Autodesk Inventor part; units mm, degrees
(part 4 of 6)
  line L2631 (12.0453, 185.408) -> (12.0771, 185.6164)
  line L2632 (12.0771, 185.6164) -> (12.1288, 185.8178)
  line L2633 (12.1288, 185.8178) -> (12.1994, 186.0107)
  line L2634 (12.1994, 186.0107) -> (12.288, 186.1941)
  line L2635 (12.288, 186.1941) -> (12.393, 186.3673)
  line L2636 (12.393, 186.3673) -> (12.514, 186.529)
  line L2637 (12.514, 186.529) -> (12.6495, 186.6782)
  line L2638 (12.6495, 186.6782) -> (12.7987, 186.8137)
  line L2639 (12.7987, 186.8137) -> (12.9603, 186.9345)
  line L2640 (12.9603, 186.9345) -> (13.1334, 187.0397)
  line L2641 (13.1334, 187.0397) -> (13.317, 187.1281)
  line L2642 (13.317, 187.1281) -> (13.5099, 187.1987)
  line L2643 (13.5099, 187.1987) -> (13.7111, 187.2506)
  line L2644 (13.7111, 187.2506) -> (13.9197, 187.2823)
  line L2645 (13.9197, 187.2823) -> (14.1344, 187.2931)
  line L2646 (14.1344, 187.2931) -> (14.3492, 187.2823)
  line L2647 (14.3492, 187.2823) -> (14.5576, 187.2506)
  line L2648 (14.5576, 187.2506) -> (14.759, 187.1987)
  line L2649 (14.759, 187.1987) -> (14.9519, 187.1281)
  line L2650 (14.9519, 187.1281) -> (15.1355, 187.0397)
  line L2651 (15.1355, 187.0397) -> (15.3086, 186.9345)
  line L2652 (15.3086, 186.9345) -> (15.4702, 186.8137)
  line L2653 (15.4702, 186.8137) -> (15.6194, 186.6782)
  line L2654 (15.6194, 186.6782) -> (15.7549, 186.529)
  line L2655 (15.7549, 186.529) -> (15.8759, 186.3673)
  line L2656 (15.8759, 186.3673) -> (15.9809, 186.1941)
  line L2657 (15.9809, 186.1941) -> (16.0695, 186.0107)
  line L2658 (16.0695, 186.0107) -> (16.1401, 185.8178)
  line L2659 (16.1401, 185.8178) -> (16.1918, 185.6164)
  line L2660 (16.1918, 185.6164) -> (16.2236, 185.408)
  line L2661 (16.2236, 185.408) -> (16.2345, 185.1932)
  line L2662 (16.2345, 185.1932) -> (16.2236, 184.9785)
  line L2663 (16.2236, 184.9785) -> (16.1918, 184.7699)
  line L2664 (16.1918, 184.7699) -> (16.1401, 184.5688)
  line L2665 (16.1401, 184.5688) -> (16.0695, 184.3758)
  line L2666 (16.0695, 184.3758) -> (15.9809, 184.1922)
  line L2667 (15.9809, 184.1922) -> (15.8759, 184.0191)
  line L2668 (15.8759, 184.0191) -> (15.7549, 183.8573)
  line L2669 (15.7549, 183.8573) -> (15.6194, 183.7083)
  line L2670 (15.6194, 183.7083) -> (15.4702, 183.5728)
  line L2671 (15.4702, 183.5728) -> (15.3086, 183.4519)
  line L2672 (15.3086, 183.4519) -> (15.1355, 183.3466)
  line L2673 (15.1355, 183.3466) -> (14.9519, 183.2582)
  line L2674 (14.9519, 183.2582) -> (14.759, 183.1876)
  line L2675 (14.759, 183.1876) -> (14.5576, 183.1359)
  line L2676 (14.5576, 183.1359) -> (14.3492, 183.1041)
  line L2677 (14.3492, 183.1041) -> (14.1344, 183.0932)
  line L2678 (14.1344, 183.0932) -> (13.9197, 183.1041)
  line L2679 (13.9197, 183.1041) -> (13.7111, 183.1359)
  line L2680 (13.7111, 183.1359) -> (13.5099, 183.1876)
  line L2681 (13.5099, 183.1876) -> (13.317, 183.2582)
  line L2682 (13.317, 183.2582) -> (13.1334, 183.3466)
  line L2683 (13.1334, 183.3466) -> (12.9603, 183.4519)
  line L2684 (12.9603, 183.4519) -> (12.7987, 183.5728)
  line L2685 (12.7987, 183.5728) -> (12.6495, 183.7083)
  line L2686 (12.6495, 183.7083) -> (12.514, 183.8573)
  line L2687 (12.514, 183.8573) -> (12.393, 184.0191)
  line L2688 (12.393, 184.0191) -> (12.288, 184.1922)
  line L2689 (12.288, 184.1922) -> (12.1994, 184.3758)
  line L2690 (12.1994, 184.3758) -> (12.1288, 184.5688)
  line L2691 (12.1288, 184.5688) -> (12.0771, 184.7699)
  line L2692 (12.0771, 184.7699) -> (12.0453, 184.9785)
  line L2693 (12.0453, 184.9785) -> (12.0344, 185.1932)
  spline S7 degree 3 poles (8.728, 122.2027) (8.728, 119.9937) (10.5189, 118.2029) (12.7281, 118.2029) knots 0 0 0 0 1 1 1 1
  line L2694 (8.728, 122.2027) -> (8.728, 119.9937) construction
  line L2695 (8.728, 119.9937) -> (10.5189, 118.2029) construction
  line L2696 (10.5189, 118.2029) -> (12.7281, 118.2029) construction
  line L2697 (12.7281, 118.2029) -> (42.201, 118.2029)
  spline S8 degree 3 poles (42.201, 118.2029) (44.4102, 118.2029) (46.201, 119.9937) (46.201, 122.2027) knots 2 2 2 2 3 3 3 3
  line L2698 (42.201, 118.2029) -> (44.4102, 118.2029) construction
  line L2699 (44.4102, 118.2029) -> (46.201, 119.9937) construction
  line L2700 (46.201, 119.9937) -> (46.201, 122.2027) construction
  line L2701 (46.201, 122.2027) -> (46.201, 175.1969)
  spline S9 degree 3 poles (46.201, 175.1969) (46.201, 177.4059) (44.4102, 179.1968) (42.201, 179.1968) knots 4 4 4 4 5 5 5 5
  line L2702 (46.201, 175.1969) -> (46.201, 177.4059) construction
  line L2703 (46.201, 177.4059) -> (44.4102, 179.1968) construction
  line L2704 (44.4102, 179.1968) -> (42.201, 179.1968) construction
  line L2705 (42.201, 179.1968) -> (12.7281, 179.1968)
  spline S10 degree 3 poles (12.7281, 179.1968) (10.5189, 179.1968) (8.728, 177.4059) (8.728, 175.1969) knots 6 6 6 6 7 7 7 7
  line L2706 (12.7281, 179.1968) -> (10.5189, 179.1968) construction
  line L2707 (10.5189, 179.1968) -> (8.728, 177.4059) construction
  line L2708 (8.728, 177.4059) -> (8.728, 175.1969) construction
  line L2709 (8.728, 175.1969) -> (8.728, 122.2027)
  line L2710 (95.0822, 167.9448) -> (83.8302, 179.1968)
  line L2711 (83.8302, 179.1968) -> (61.6093, 179.1968)
  spline S11 degree 3 poles (61.6093, 179.1968) (59.4002, 179.1968) (57.6092, 177.4059) (57.6092, 175.1969) knots 2 2 2 2 3 3 3 3
  line L2712 (61.6093, 179.1968) -> (59.4002, 179.1968) construction
  line L2713 (59.4002, 179.1968) -> (57.6092, 177.4059) construction
  line L2714 (57.6092, 177.4059) -> (57.6092, 175.1969) construction
  line L2715 (57.6092, 175.1969) -> (57.6092, 122.2027)
  spline S12 degree 3 poles (57.6092, 122.2027) (57.6092, 119.9937) (59.4002, 118.2029) (61.6093, 118.2029) knots 4 4 4 4 5 5 5 5
  line L2716 (57.6092, 122.2027) -> (57.6092, 119.9937) construction
  line L2717 (57.6092, 119.9937) -> (59.4002, 118.2029) construction
  line L2718 (59.4002, 118.2029) -> (61.6093, 118.2029) construction
  line L2719 (61.6093, 118.2029) -> (91.0823, 118.2029)
  spline S13 degree 3 poles (91.0823, 118.2029) (93.2915, 118.2029) (95.0822, 119.9937) (95.0822, 122.2027) knots 6 6 6 6 7 7 7 7
  line L2720 (91.0823, 118.2029) -> (93.2915, 118.2029) construction
  line L2721 (93.2915, 118.2029) -> (95.0822, 119.9937) construction
  line L2722 (95.0822, 119.9937) -> (95.0822, 122.2027) construction
  line L2723 (95.0822, 122.2027) -> (95.0822, 167.9448)
  spline S14 degree 3 poles (98.6277, 167.2363) (98.6277, 164.4749) (100.8664, 162.2363) (103.6278, 162.2363) knots 0 0 0 0 1 1 1 1
  line L2724 (98.6277, 167.2363) -> (98.6277, 164.4749) construction
  line L2725 (98.6277, 164.4749) -> (100.8664, 162.2363) construction
  line L2726 (100.8664, 162.2363) -> (103.6278, 162.2363) construction
  line L2727 (103.6278, 162.2363) -> (106.6278, 162.2363)
  spline S15 degree 3 poles (106.6278, 162.2363) (109.3894, 162.2363) (111.6276, 164.4749) (111.6276, 167.2363) knots 2 2 2 2 3 3 3 3
  line L2728 (106.6278, 162.2363) -> (109.3894, 162.2363) construction
  line L2729 (109.3894, 162.2363) -> (111.6276, 164.4749) construction
  line L2730 (111.6276, 164.4749) -> (111.6276, 167.2363) construction
  line L2731 (111.6276, 167.2363) -> (111.6276, 174.2373)
  spline S16 degree 3 poles (111.6276, 174.2373) (111.6276, 176.9987) (109.3894, 179.2373) (106.6278, 179.2373) knots 4 4 4 4 5 5 5 5
  line L2732 (111.6276, 174.2373) -> (111.6276, 176.9987) construction
  line L2733 (111.6276, 176.9987) -> (109.3894, 179.2373) construction
  line L2734 (109.3894, 179.2373) -> (106.6278, 179.2373) construction
  line L2735 (106.6278, 179.2373) -> (103.6278, 179.2373)
  spline S17 degree 3 poles (103.6278, 179.2373) (100.8664, 179.2373) (98.6277, 176.9987) (98.6277, 174.2373) knots 6 6 6 6 7 7 7 7
  line L2736 (103.6278, 179.2373) -> (100.8664, 179.2373) construction
  line L2737 (100.8664, 179.2373) -> (98.6277, 176.9987) construction
  line L2738 (98.6277, 176.9987) -> (98.6277, 174.2373) construction
  line L2739 (98.6277, 174.2373) -> (98.6277, 167.2363)
  spline S18 degree 3 poles (98.6277, 145.2363) (98.6277, 142.475) (100.8664, 140.2364) (103.6278, 140.2364) knots 0 0 0 0 1 1 1 1
  line L2740 (98.6277, 145.2363) -> (98.6277, 142.475) construction
  line L2741 (98.6277, 142.475) -> (100.8664, 140.2364) construction
  line L2742 (100.8664, 140.2364) -> (103.6278, 140.2364) construction
  line L2743 (103.6278, 140.2364) -> (106.6278, 140.2364)
  spline S19 degree 3 poles (106.6278, 140.2364) (109.3894, 140.2364) (111.6276, 142.475) (111.6276, 145.2363) knots 2 2 2 2 3 3 3 3
  line L2744 (106.6278, 140.2364) -> (109.3894, 140.2364) construction
  line L2745 (109.3894, 140.2364) -> (111.6276, 142.475) construction
  line L2746 (111.6276, 142.475) -> (111.6276, 145.2363) construction
  line L2747 (111.6276, 145.2363) -> (111.6276, 152.2374)
  spline S20 degree 3 poles (111.6276, 152.2374) (111.6276, 154.9988) (109.3894, 157.2373) (106.6278, 157.2373) knots 4 4 4 4 5 5 5 5
  line L2748 (111.6276, 152.2374) -> (111.6276, 154.9988) construction
  line L2749 (111.6276, 154.9988) -> (109.3894, 157.2373) construction
  line L2750 (109.3894, 157.2373) -> (106.6278, 157.2373) construction
  line L2751 (106.6278, 157.2373) -> (103.6278, 157.2373)
  spline S21 degree 3 poles (103.6278, 157.2373) (100.8664, 157.2373) (98.6277, 154.9988) (98.6277, 152.2374) knots 6 6 6 6 7 7 7 7
  line L2752 (103.6278, 157.2373) -> (100.8664, 157.2373) construction
  line L2753 (100.8664, 157.2373) -> (98.6277, 154.9988) construction
  line L2754 (98.6277, 154.9988) -> (98.6277, 152.2374) construction
  line L2755 (98.6277, 152.2374) -> (98.6277, 145.2363)
  spline S22 degree 3 poles (98.6277, 123.2362) (98.6277, 120.475) (100.8664, 118.2364) (103.6278, 118.2364) knots 0 0 0 0 1 1 1 1
  line L2756 (98.6277, 123.2362) -> (98.6277, 120.475) construction
  line L2757 (98.6277, 120.475) -> (100.8664, 118.2364) construction
  line L2758 (100.8664, 118.2364) -> (103.6278, 118.2364) construction
  line L2759 (103.6278, 118.2364) -> (106.6278, 118.2364)
  spline S23 degree 3 poles (106.6278, 118.2364) (109.3894, 118.2364) (111.6276, 120.475) (111.6276, 123.2362) knots 2 2 2 2 3 3 3 3
  line L2760 (106.6278, 118.2364) -> (109.3894, 118.2364) construction
  line L2761 (109.3894, 118.2364) -> (111.6276, 120.475) construction
  line L2762 (111.6276, 120.475) -> (111.6276, 123.2362) construction
  line L2763 (111.6276, 123.2362) -> (111.6276, 130.2374)
  spline S24 degree 3 poles (111.6276, 130.2374) (111.6276, 132.9986) (109.3894, 135.2372) (106.6278, 135.2372) knots 4 4 4 4 5 5 5 5
  line L2764 (111.6276, 130.2374) -> (111.6276, 132.9986) construction
  line L2765 (111.6276, 132.9986) -> (109.3894, 135.2372) construction
  line L2766 (109.3894, 135.2372) -> (106.6278, 135.2372) construction
  line L2767 (106.6278, 135.2372) -> (103.6278, 135.2372)
  spline S25 degree 3 poles (103.6278, 135.2372) (100.8664, 135.2372) (98.6277, 132.9986) (98.6277, 130.2374) knots 6 6 6 6 7 7 7 7
  line L2768 (103.6278, 135.2372) -> (100.8664, 135.2372) construction
  line L2769 (100.8664, 135.2372) -> (98.6277, 132.9986) construction
  line L2770 (98.6277, 132.9986) -> (98.6277, 130.2374) construction
  line L2771 (98.6277, 130.2374) -> (98.6277, 123.2362)
  line L2772 (115.0824, 123.8495) -> (115.0896, 123.569)
  line L2773 (115.0896, 123.569) -> (115.1124, 123.2907)
  line L2774 (115.1124, 123.2907) -> (115.2009, 122.7415)
  line L2775 (115.2009, 122.7415) -> (115.3466, 122.2051)
  line L2776 (115.3466, 122.2051) -> (115.5478, 121.6859)
  line L2777 (115.5478, 121.6859) -> (115.8024, 121.1874)
  line L2778 (115.8024, 121.1874) -> (116.1094, 120.713)
  line L2779 (116.1094, 120.713) -> (116.467, 120.2666)
  line L2780 (116.467, 120.2666) -> (116.8731, 119.8521)
  line L2781 (116.8731, 119.8521) -> (117.3217, 119.4766)
  line L2782 (117.3217, 119.4766) -> (117.8044, 119.1462)
  line L2783 (117.8044, 119.1462) -> (118.3173, 118.8623)
  line L2784 (118.3173, 118.8623) -> (118.8568, 118.6267)
  line L2785 (118.8568, 118.6267) -> (119.4184, 118.4407)
  line L2786 (119.4184, 118.4407) -> (119.9982, 118.306)
  line L2787 (119.9982, 118.306) -> (120.5921, 118.224)
  line L2788 (120.5921, 118.224) -> (121.1967, 118.1964)
  line L2789 (121.1967, 118.1964) -> (195.3128, 118.1964)
  line L2790 (195.3128, 118.1964) -> (195.9174, 118.224)
  line L2791 (195.9174, 118.224) -> (196.5113, 118.306)
  line L2792 (196.5113, 118.306) -> (197.0912, 118.4407)
  line L2793 (197.0912, 118.4407) -> (197.6527, 118.6267)
  line L2794 (197.6527, 118.6267) -> (198.1922, 118.8623)
  line L2795 (198.1922, 118.8623) -> (198.7052, 119.1462)
  line L2796 (198.7052, 119.1462) -> (199.1878, 119.4766)
  line L2797 (199.1878, 119.4766) -> (199.6364, 119.8521)
  line L2798 (199.6364, 119.8521) -> (200.0426, 120.2666)
  line L2799 (200.0426, 120.2666) -> (200.4002, 120.713)
  line L2800 (200.4002, 120.713) -> (200.7071, 121.1874)
  line L2801 (200.7071, 121.1874) -> (200.9617, 121.6859)
  line L2802 (200.9617, 121.6859) -> (201.1629, 122.2051)
  line L2803 (201.1629, 122.2051) -> (201.3086, 122.7415)
  line L2804 (201.3086, 122.7415) -> (201.3975, 123.2907)
  line L2805 (201.3975, 123.2907) -> (201.4199, 123.569)
  line L2806 (201.4199, 123.569) -> (201.4272, 123.8495)
  line L2807 (201.4272, 123.8495) -> (201.4272, 173.5424)
  line L2808 (201.4272, 173.5424) -> (201.4199, 173.8226)
  line L2809 (201.4199, 173.8226) -> (201.3975, 174.101)
  line L2810 (201.3975, 174.101) -> (201.3086, 174.6503)
  line L2811 (201.3086, 174.6503) -> (201.1629, 175.1864)
  line L2812 (201.1629, 175.1864) -> (200.9617, 175.7056)
  line L2813 (200.9617, 175.7056) -> (200.7071, 176.2042)
  line L2814 (200.7071, 176.2042) -> (200.4002, 176.6786)
  line L2815 (200.4002, 176.6786) -> (200.0426, 177.1249)
  line L2816 (200.0426, 177.1249) -> (199.6364, 177.5396)
  line L2817 (199.6364, 177.5396) -> (199.1878, 177.9151)
  line L2818 (199.1878, 177.9151) -> (198.7052, 178.2456)
  line L2819 (198.7052, 178.2456) -> (198.1922, 178.5293)
  line L2820 (198.1922, 178.5293) -> (197.6527, 178.765)
  line L2821 (197.6527, 178.765) -> (197.0912, 178.951)
  line L2822 (197.0912, 178.951) -> (196.5113, 179.0857)
  line L2823 (196.5113, 179.0857) -> (195.9174, 179.1677)
  line L2824 (195.9174, 179.1677) -> (195.3128, 179.1953)
  line L2825 (195.3128, 179.1953) -> (121.1967, 179.1953)
  line L2826 (121.1967, 179.1953) -> (120.5921, 179.1677)
  line L2827 (120.5921, 179.1677) -> (119.9982, 179.0857)
  line L2828 (119.9982, 179.0857) -> (119.4184, 178.951)
  line L2829 (119.4184, 178.951) -> (118.8568, 178.765)
  line L2830 (118.8568, 178.765) -> (118.3173, 178.5293)
  line L2831 (118.3173, 178.5293) -> (117.8044, 178.2456)
  line L2832 (117.8044, 178.2456) -> (117.3217, 177.9151)
  line L2833 (117.3217, 177.9151) -> (116.8731, 177.5396)
  line L2834 (116.8731, 177.5396) -> (116.467, 177.1249)
  line L2835 (116.467, 177.1249) -> (116.1094, 176.6786)
  line L2836 (116.1094, 176.6786) -> (115.8024, 176.2042)
  line L2837 (115.8024, 176.2042) -> (115.5478, 175.7056)
  line L2838 (115.5478, 175.7056) -> (115.3466, 175.1864)
  line L2839 (115.3466, 175.1864) -> (115.2009, 174.6503)
  line L2840 (115.2009, 174.6503) -> (115.1124, 174.101)
  line L2841 (115.1124, 174.101) -> (115.0896, 173.8226)
  line L2842 (115.0896, 173.8226) -> (115.0824, 173.5424)
  line L2843 (115.0824, 173.5424) -> (115.0824, 123.8495)
  line L2844 (93.5268, 176.2439) -> (93.535, 176.4075)
  line L2845 (93.535, 176.4075) -> (93.5593, 176.5663)
  line L2846 (93.5593, 176.5663) -> (93.5988, 176.7196)
  line L2847 (93.5988, 176.7196) -> (93.6525, 176.8666)
  line L2848 (93.6525, 176.8666) -> (93.7199, 177.0064)
  line L2849 (93.7199, 177.0064) -> (93.8, 177.1384)
  line L2850 (93.8, 177.1384) -> (93.9955, 177.3752)
  line L2851 (93.9955, 177.3752) -> (94.2321, 177.5706)
  line L2852 (94.2321, 177.5706) -> (94.3641, 177.6507)
  line L2853 (94.3641, 177.6507) -> (94.504, 177.718)
  line L2854 (94.504, 177.718) -> (94.6509, 177.7719)
  line L2855 (94.6509, 177.7719) -> (94.8044, 177.8114)
  line L2856 (94.8044, 177.8114) -> (94.9632, 177.8355)
  line L2857 (94.9632, 177.8355) -> (95.1268, 177.8438)
  line L2858 (95.1268, 177.8438) -> (95.2903, 177.8355)
  line L2859 (95.2903, 177.8355) -> (95.4493, 177.8114)
  line L2860 (95.4493, 177.8114) -> (95.6026, 177.7719)
  line L2861 (95.6026, 177.7719) -> (95.7495, 177.718)
  line L2862 (95.7495, 177.718) -> (95.8894, 177.6507)
  line L2863 (95.8894, 177.6507) -> (96.0214, 177.5706)
  line L2864 (96.0214, 177.5706) -> (96.2582, 177.3752)
  line L2865 (96.2582, 177.3752) -> (96.4535, 177.1384)
  line L2866 (96.4535, 177.1384) -> (96.5336, 177.0064)
  line L2867 (96.5336, 177.0064) -> (96.601, 176.8666)
  line L2868 (96.601, 176.8666) -> (96.6549, 176.7196)
  line L2869 (96.6549, 176.7196) -> (96.6942, 176.5663)
  line L2870 (96.6942, 176.5663) -> (96.7185, 176.4075)
  line L2871 (96.7185, 176.4075) -> (96.7267, 176.2439)
  line L2872 (96.7267, 176.2439) -> (96.7185, 176.0802)
  line L2873 (96.7185, 176.0802) -> (96.6942, 175.9214)
  line L2874 (96.6942, 175.9214) -> (96.6549, 175.7681)
  line L2875 (96.6549, 175.7681) -> (96.601, 175.621)
  line L2876 (96.601, 175.621) -> (96.5336, 175.4811)
  line L2877 (96.5336, 175.4811) -> (96.4535, 175.3493)
  line L2878 (96.4535, 175.3493) -> (96.2582, 175.1125)
  line L2879 (96.2582, 175.1125) -> (96.0214, 174.9171)
  line L2880 (96.0214, 174.9171) -> (95.8894, 174.8369)
  line L2881 (95.8894, 174.8369) -> (95.7495, 174.7695)
  line L2882 (95.7495, 174.7695) -> (95.6026, 174.7158)
  line L2883 (95.6026, 174.7158) -> (95.4493, 174.6763)
  line L2884 (95.4493, 174.6763) -> (95.2903, 174.652)
  line L2885 (95.2903, 174.652) -> (95.1268, 174.6438)
  line L2886 (95.1268, 174.6438) -> (94.9632, 174.652)
  line L2887 (94.9632, 174.652) -> (94.8044, 174.6763)
  line L2888 (94.8044, 174.6763) -> (94.6509, 174.7158)
  line L2889 (94.6509, 174.7158) -> (94.504, 174.7695)
  line L2890 (94.504, 174.7695) -> (94.3641, 174.8369)
  line L2891 (94.3641, 174.8369) -> (94.2321, 174.9171)
  line L2892 (94.2321, 174.9171) -> (93.9955, 175.1125)
  line L2893 (93.9955, 175.1125) -> (93.8, 175.3493)
  line L2894 (93.8, 175.3493) -> (93.7199, 175.4811)
  line L2895 (93.7199, 175.4811) -> (93.6525, 175.621)
  line L2896 (93.6525, 175.621) -> (93.5988, 175.7681)
  line L2897 (93.5988, 175.7681) -> (93.5593, 175.9214)
  line L2898 (93.5593, 175.9214) -> (93.535, 176.0802)
  line L2899 (93.535, 176.0802) -> (93.5268, 176.2439)
  spline S26 degree 3 poles (49.2468, 171.5606) (49.2468, 170.18) (50.3661, 169.0607) (51.7467, 169.0607) knots 0 0 0 0 1 1 1 1
  line L2900 (49.2468, 171.5606) -> (49.2468, 170.18) construction
  line L2901 (49.2468, 170.18) -> (50.3661, 169.0607) construction
  line L2902 (50.3661, 169.0607) -> (51.7467, 169.0607) construction
  line L2903 (51.7467, 169.0607) -> (52.6047, 169.0607)
  spline S27 degree 3 poles (52.6047, 169.0607) (53.9855, 169.0607) (55.1048, 170.18) (55.1048, 171.5606) knots 2 2 2 2 3 3 3 3
  line L2904 (52.6047, 169.0607) -> (53.9855, 169.0607) construction
  line L2905 (53.9855, 169.0607) -> (55.1048, 170.18) construction
  line L2906 (55.1048, 170.18) -> (55.1048, 171.5606) construction
  line L2907 (55.1048, 171.5606) -> (55.1048, 176.5606)
  spline S28 degree 3 poles (55.1048, 176.5606) (55.1048, 177.9414) (53.9855, 179.0607) (52.6047, 179.0607) knots 4 4 4 4 5 5 5 5
  line L2908 (55.1048, 176.5606) -> (55.1048, 177.9414) construction
  line L2909 (55.1048, 177.9414) -> (53.9855, 179.0607) construction
  line L2910 (53.9855, 179.0607) -> (52.6047, 179.0607) construction
  line L2911 (52.6047, 179.0607) -> (51.7467, 179.0607)
  spline S29 degree 3 poles (51.7467, 179.0607) (50.3661, 179.0607) (49.2468, 177.9414) (49.2468, 176.5606) knots 6 6 6 6 7 7 7 7
  line L2912 (51.7467, 179.0607) -> (50.3661, 179.0607) construction
  line L2913 (50.3661, 179.0607) -> (49.2468, 177.9414) construction
  line L2914 (49.2468, 177.9414) -> (49.2468, 176.5606) construction
  line L2915 (49.2468, 176.5606) -> (49.2468, 171.5606)
  spline S30 degree 3 poles (49.2468, 158.8606) (49.2468, 157.48) (50.3661, 156.3607) (51.7467, 156.3607) knots 0 0 0 0 1 1 1 1
  line L2916 (49.2468, 158.8606) -> (49.2468, 157.48) construction
  line L2917 (49.2468, 157.48) -> (50.3661, 156.3607) construction
  line L2918 (50.3661, 156.3607) -> (51.7467, 156.3607) construction
  line L2919 (51.7467, 156.3607) -> (52.6047, 156.3607)
  spline S31 degree 3 poles (52.6047, 156.3607) (53.9855, 156.3607) (55.1048, 157.48) (55.1048, 158.8606) knots 2 2 2 2 3 3 3 3
  line L2920 (52.6047, 156.3607) -> (53.9855, 156.3607) construction
  line L2921 (53.9855, 156.3607) -> (55.1048, 157.48) construction
  line L2922 (55.1048, 157.48) -> (55.1048, 158.8606) construction
  line L2923 (55.1048, 158.8606) -> (55.1048, 163.8606)
  spline S32 degree 3 poles (55.1048, 163.8606) (55.1048, 165.2414) (53.9855, 166.3607) (52.6047, 166.3607) knots 4 4 4 4 5 5 5 5
  line L2924 (55.1048, 163.8606) -> (55.1048, 165.2414) construction
  line L2925 (55.1048, 165.2414) -> (53.9855, 166.3607) construction
  line L2926 (53.9855, 166.3607) -> (52.6047, 166.3607) construction
  line L2927 (52.6047, 166.3607) -> (51.7467, 166.3607)
  spline S33 degree 3 poles (51.7467, 166.3607) (50.3661, 166.3607) (49.2468, 165.2414) (49.2468, 163.8606) knots 6 6 6 6 7 7 7 7
  line L2928 (51.7467, 166.3607) -> (50.3661, 166.3607) construction
  line L2929 (50.3661, 166.3607) -> (49.2468, 165.2414) construction
  line L2930 (49.2468, 165.2414) -> (49.2468, 163.8606) construction
  line L2931 (49.2468, 163.8606) -> (49.2468, 158.8606)
  spline S34 degree 3 poles (49.2468, 146.1606) (49.2468, 144.7798) (50.3661, 143.6605) (51.7467, 143.6605) knots 0 0 0 0 1 1 1 1
  line L2932 (49.2468, 146.1606) -> (49.2468, 144.7798) construction
  line L2933 (49.2468, 144.7798) -> (50.3661, 143.6605) construction
  line L2934 (50.3661, 143.6605) -> (51.7467, 143.6605) construction
  line L2935 (51.7467, 143.6605) -> (52.6047, 143.6605)
  spline S35 degree 3 poles (52.6047, 143.6605) (53.9855, 143.6605) (55.1048, 144.7798) (55.1048, 146.1606) knots 2 2 2 2 3 3 3 3
  line L2936 (52.6047, 143.6605) -> (53.9855, 143.6605) construction
  line L2937 (53.9855, 143.6605) -> (55.1048, 144.7798) construction
  line L2938 (55.1048, 144.7798) -> (55.1048, 146.1606) construction
  line L2939 (55.1048, 146.1606) -> (55.1048, 151.1606)
  spline S36 degree 3 poles (55.1048, 151.1606) (55.1048, 152.5414) (53.9855, 153.6607) (52.6047, 153.6607) knots 4 4 4 4 5 5 5 5
  line L2940 (55.1048, 151.1606) -> (55.1048, 152.5414) construction
  line L2941 (55.1048, 152.5414) -> (53.9855, 153.6607) construction
  line L2942 (53.9855, 153.6607) -> (52.6047, 153.6607) construction
  line L2943 (52.6047, 153.6607) -> (51.7467, 153.6607)
  spline S37 degree 3 poles (51.7467, 153.6607) (50.3661, 153.6607) (49.2468, 152.5414) (49.2468, 151.1606) knots 6 6 6 6 7 7 7 7
  line L2944 (51.7467, 153.6607) -> (50.3661, 153.6607) construction
  line L2945 (50.3661, 153.6607) -> (49.2468, 152.5414) construction
  line L2946 (49.2468, 152.5414) -> (49.2468, 151.1606) construction
  line L2947 (49.2468, 151.1606) -> (49.2468, 146.1606)
  spline S38 degree 3 poles (49.2468, 133.4606) (49.2468, 132.0798) (50.3661, 130.9605) (51.7467, 130.9605) knots 0 0 0 0 1 1 1 1
  line L2948 (49.2468, 133.4606) -> (49.2468, 132.0798) construction
  line L2949 (49.2468, 132.0798) -> (50.3661, 130.9605) construction
  line L2950 (50.3661, 130.9605) -> (51.7467, 130.9605) construction
  line L2951 (51.7467, 130.9605) -> (52.6047, 130.9605)
  spline S39 degree 3 poles (52.6047, 130.9605) (53.9855, 130.9605) (55.1048, 132.0798) (55.1048, 133.4606) knots 2 2 2 2 3 3 3 3
  line L2952 (52.6047, 130.9605) -> (53.9855, 130.9605) construction
  line L2953 (53.9855, 130.9605) -> (55.1048, 132.0798) construction
  line L2954 (55.1048, 132.0798) -> (55.1048, 133.4606) construction
  line L2955 (55.1048, 133.4606) -> (55.1048, 138.4608)
  spline S40 degree 3 poles (55.1048, 138.4608) (55.1048, 139.8412) (53.9855, 140.9606) (52.6047, 140.9606) knots 4 4 4 4 5 5 5 5
  line L2956 (55.1048, 138.4608) -> (55.1048, 139.8412) construction
  line L2957 (55.1048, 139.8412) -> (53.9855, 140.9606) construction
  line L2958 (53.9855, 140.9606) -> (52.6047, 140.9606) construction
  line L2959 (52.6047, 140.9606) -> (51.7467, 140.9606)
  spline S41 degree 3 poles (51.7467, 140.9606) (50.3661, 140.9606) (49.2468, 139.8412) (49.2468, 138.4608) knots 6 6 6 6 7 7 7 7
  line L2960 (51.7467, 140.9606) -> (50.3661, 140.9606) construction
  line L2961 (50.3661, 140.9606) -> (49.2468, 139.8412) construction
  line L2962 (49.2468, 139.8412) -> (49.2468, 138.4608) construction
  line L2963 (49.2468, 138.4608) -> (49.2468, 133.4606)
  spline S42 degree 3 poles (49.2468, 120.7606) (49.2468, 119.3798) (50.3661, 118.2605) (51.7467, 118.2605) knots 0 0 0 0 1 1 1 1
  line L2964 (49.2468, 120.7606) -> (49.2468, 119.3798) construction
  line L2965 (49.2468, 119.3798) -> (50.3661, 118.2605) construction
  line L2966 (50.3661, 118.2605) -> (51.7467, 118.2605) construction
  line L2967 (51.7467, 118.2605) -> (52.6047, 118.2605)
  spline S43 degree 3 poles (52.6047, 118.2605) (53.9855, 118.2605) (55.1048, 119.3798) (55.1048, 120.7606) knots 2 2 2 2 3 3 3 3
  line L2968 (52.6047, 118.2605) -> (53.9855, 118.2605) construction
  line L2969 (53.9855, 118.2605) -> (55.1048, 119.3798) construction
  line L2970 (55.1048, 119.3798) -> (55.1048, 120.7606) construction
  line L2971 (55.1048, 120.7606) -> (55.1048, 125.7608)
  spline S44 degree 3 poles (55.1048, 125.7608) (55.1048, 127.1412) (53.9855, 128.2606) (52.6047, 128.2606) knots 4 4 4 4 5 5 5 5
  line L2972 (55.1048, 125.7608) -> (55.1048, 127.1412) construction
  line L2973 (55.1048, 127.1412) -> (53.9855, 128.2606) construction
  line L2974 (53.9855, 128.2606) -> (52.6047, 128.2606) construction
  line L2975 (52.6047, 128.2606) -> (51.7467, 128.2606)
  spline S45 degree 3 poles (51.7467, 128.2606) (50.3661, 128.2606) (49.2468, 127.1412) (49.2468, 125.7608) knots 6 6 6 6 7 7 7 7
  line L2976 (51.7467, 128.2606) -> (50.3661, 128.2606) construction
  line L2977 (50.3661, 128.2606) -> (49.2468, 127.1412) construction
  line L2978 (49.2468, 127.1412) -> (49.2468, 125.7608) construction
  line L2979 (49.2468, 125.7608) -> (49.2468, 120.7606)
  spline S46 degree 3 poles (212.1359, 137.696) (212.1359, 135.4866) (213.9266, 133.6959) (216.1356, 133.6959) knots 0 0 0 0 1 1 1 1
  line L2980 (212.1359, 137.696) -> (212.1359, 135.4866) construction
  line L2981 (212.1359, 135.4866) -> (213.9266, 133.6959) construction
  line L2982 (213.9266, 133.6959) -> (216.1356, 133.6959) construction
  line L2983 (216.1356, 133.6959) -> (234.1359, 133.6959)
  spline S47 degree 3 poles (234.1359, 133.6959) (236.3449, 133.6959) (238.1357, 135.4866) (238.1357, 137.696) knots 2 2 2 2 3 3 3 3
  line L2984 (234.1359, 133.6959) -> (236.3449, 133.6959) construction
  line L2985 (236.3449, 133.6959) -> (238.1357, 135.4866) construction
  line L2986 (238.1357, 135.4866) -> (238.1357, 137.696) construction
  line L2987 (238.1357, 137.696) -> (238.1357, 159.6959)
  spline S48 degree 3 poles (238.1357, 159.6959) (238.1357, 161.905) (236.3449, 163.6958) (234.1359, 163.6958) knots 4 4 4 4 5 5 5 5
  line L2988 (238.1357, 159.6959) -> (238.1357, 161.905) construction
  line L2989 (238.1357, 161.905) -> (236.3449, 163.6958) construction
  line L2990 (236.3449, 163.6958) -> (234.1359, 163.6958) construction
  line L2991 (234.1359, 163.6958) -> (216.1356, 163.6958)
  spline S49 degree 3 poles (216.1356, 163.6958) (213.9266, 163.6958) (212.1359, 161.905) (212.1359, 159.6959) knots 6 6 6 6 7 7 7 7
  line L2992 (216.1356, 163.6958) -> (213.9266, 163.6958) construction
  line L2993 (213.9266, 163.6958) -> (212.1359, 161.905) construction
  line L2994 (212.1359, 161.905) -> (212.1359, 159.6959) construction
  line L2995 (212.1359, 159.6959) -> (212.1359, 137.696)
  line L2996 (219.1274, 202.2026) -> (219.1349, 202.5113)
  line L2997 (219.1349, 202.5113) -> (219.1584, 202.816)
  line L2998 (219.1584, 202.816) -> (219.1963, 203.1163)
  line L2999 (219.1963, 203.1163) -> (219.2493, 203.4119)
  line L3000 (219.2493, 203.4119) -> (219.3971, 203.9869)
  line L3001 (219.3971, 203.9869) -> (219.5987, 204.5381)
  line L3002 (219.5987, 204.5381) -> (219.8515, 205.0626)
  line L3003 (219.8515, 205.0626) -> (220.1519, 205.5573)
  line L3004 (220.1519, 205.5573) -> (220.4975, 206.0191)
  line L3005 (220.4975, 206.0191) -> (220.8847, 206.4453)
  line L3006 (220.8847, 206.4453) -> (221.3109, 206.8325)
  line L3007 (221.3109, 206.8325) -> (221.7725, 207.1779)
  line L3008 (221.7725, 207.1779) -> (222.2672, 207.4785)
  line L3009 (222.2672, 207.4785) -> (222.7919, 207.731)
  line L3010 (222.7919, 207.731) -> (223.3431, 207.9329)
  line L3011 (223.3431, 207.9329) -> (223.9181, 208.0807)
  line L3012 (223.9181, 208.0807) -> (224.2134, 208.1334)
  line L3013 (224.2134, 208.1334) -> (224.5138, 208.1716)
  line L3014 (224.5138, 208.1716) -> (224.8187, 208.1947)
  line L3015 (224.8187, 208.1947) -> (225.1273, 208.2026)
  line L3016 (225.1273, 208.2026) -> (225.436, 208.1947)
  line L3017 (225.436, 208.1947) -> (225.7406, 208.1716)
  line L3018 (225.7406, 208.1716) -> (226.041, 208.1334)
  line L3019 (226.041, 208.1334) -> (226.3366, 208.0807)
  line L3020 (226.3366, 208.0807) -> (226.9116, 207.9329)
  line L3021 (226.9116, 207.9329) -> (227.4628, 207.731)
  line L3022 (227.4628, 207.731) -> (227.9871, 207.4785)
  line L3023 (227.9871, 207.4785) -> (228.4818, 207.1779)
  line L3024 (228.4818, 207.1779) -> (228.9438, 206.8325)
  line L3025 (228.9438, 206.8325) -> (229.37, 206.4453)
  line L3026 (229.37, 206.4453) -> (229.7572, 206.0191)
  line L3027 (229.7572, 206.0191) -> (230.1024, 205.5573)
  line L3028 (230.1024, 205.5573) -> (230.4032, 205.0626)
  line L3029 (230.4032, 205.0626) -> (230.6557, 204.5381)
  line L3030 (230.6557, 204.5381) -> (230.8576, 203.9869)
  line L3031 (230.8576, 203.9869) -> (231.0054, 203.4119)
  line L3032 (231.0054, 203.4119) -> (231.0581, 203.1163)
  line L3033 (231.0581, 203.1163) -> (231.0963, 202.816)
  line L3034 (231.0963, 202.816) -> (231.1194, 202.5113)
  line L3035 (231.1194, 202.5113) -> (231.1273, 202.2026)
  line L3036 (231.1273, 202.2026) -> (231.1194, 201.8938)
  line L3037 (231.1194, 201.8938) -> (231.0963, 201.5891)
  line L3038 (231.0963, 201.5891) -> (231.0581, 201.2888)
  line L3039 (231.0581, 201.2888) -> (231.0054, 200.9934)
  line L3040 (231.0054, 200.9934) -> (230.8576, 200.4184)
  line L3041 (230.8576, 200.4184) -> (230.6557, 199.8672)
  line L3042 (230.6557, 199.8672) -> (230.4032, 199.3427)
  line L3043 (230.4032, 199.3427) -> (230.1024, 198.848)
  line L3044 (230.1024, 198.848) -> (229.7572, 198.386)
  line L3045 (229.7572, 198.386) -> (229.37, 197.96)
  line L3046 (229.37, 197.96) -> (228.9438, 197.5728)
  line L3047 (228.9438, 197.5728) -> (228.4818, 197.2272)
  line L3048 (228.4818, 197.2272) -> (227.9871, 196.9268)
  line L3049 (227.9871, 196.9268) -> (227.4628, 196.6741)
  line L3050 (227.4628, 196.6741) -> (226.9116, 196.4724)
  line L3051 (226.9116, 196.4724) -> (226.3366, 196.3245)
  line L3052 (226.3366, 196.3245) -> (226.041, 196.2717)
  line L3053 (226.041, 196.2717) -> (225.7406, 196.2335)
  line L3054 (225.7406, 196.2335) -> (225.436, 196.2104)
  line L3055 (225.436, 196.2104) -> (225.1273, 196.2027)
  line L3056 (225.1273, 196.2027) -> (224.8187, 196.2104)
  line L3057 (224.8187, 196.2104) -> (224.5138, 196.2335)
  line L3058 (224.5138, 196.2335) -> (224.2134, 196.2717)
  line L3059 (224.2134, 196.2717) -> (223.9181, 196.3245)
  line L3060 (223.9181, 196.3245) -> (223.3431, 196.4724)
  line L3061 (223.3431, 196.4724) -> (222.7919, 196.6741)
  line L3062 (222.7919, 196.6741) -> (222.2672, 196.9268)
  line L3063 (222.2672, 196.9268) -> (221.7725, 197.2272)
  line L3064 (221.7725, 197.2272) -> (221.3109, 197.5728)
  line L3065 (221.3109, 197.5728) -> (220.8847, 197.96)
  line L3066 (220.8847, 197.96) -> (220.4975, 198.386)
  line L3067 (220.4975, 198.386) -> (220.1519, 198.848)
  line L3068 (220.1519, 198.848) -> (219.8515, 199.3427)
  line L3069 (219.8515, 199.3427) -> (219.5987, 199.8672)
  line L3070 (219.5987, 199.8672) -> (219.3971, 200.4184)
  line L3071 (219.3971, 200.4184) -> (219.2493, 200.9934)
  line L3072 (219.2493, 200.9934) -> (219.1963, 201.2888)
  line L3073 (219.1963, 201.2888) -> (219.1584, 201.5891)
  line L3074 (219.1584, 201.5891) -> (219.1349, 201.8938)
  line L3075 (219.1349, 201.8938) -> (219.1274, 202.2026)
  line L3076 (219.1274, 95.1987) -> (219.1349, 95.5073)
  line L3077 (219.1349, 95.5073) -> (219.1584, 95.8119)
  line L3078 (219.1584, 95.8119) -> (219.1963, 96.1123)
  line L3079 (219.1963, 96.1123) -> (219.2493, 96.4079)
  line L3080 (219.2493, 96.4079) -> (219.3971, 96.9829)
  line L3081 (219.3971, 96.9829) -> (219.5987, 97.5341)
  line L3082 (219.5987, 97.5341) -> (219.8515, 98.0584)
  line L3083 (219.8515, 98.0584) -> (220.1519, 98.5532)
  line L3084 (220.1519, 98.5532) -> (220.4975, 99.0151)
  line L3085 (220.4975, 99.0151) -> (220.8847, 99.4413)
  line L3086 (220.8847, 99.4413) -> (221.3109, 99.8285)
  line L3087 (221.3109, 99.8285) -> (221.7725, 100.1737)
  line L3088 (221.7725, 100.1737) -> (222.2672, 100.4745)
  line L3089 (222.2672, 100.4745) -> (222.7919, 100.727)
  line L3090 (222.7919, 100.727) -> (223.3431, 100.9289)
  line L3091 (223.3431, 100.9289) -> (223.9181, 101.0767)
  line L3092 (223.9181, 101.0767) -> (224.2134, 101.1294)
  line L3093 (224.2134, 101.1294) -> (224.5138, 101.1676)
  line L3094 (224.5138, 101.1676) -> (224.8187, 101.1907)
  line L3095 (224.8187, 101.1907) -> (225.1273, 101.1986)
  line L3096 (225.1273, 101.1986) -> (225.436, 101.1907)
  line L3097 (225.436, 101.1907) -> (225.7406, 101.1676)
  line L3098 (225.7406, 101.1676) -> (226.041, 101.1294)
  line L3099 (226.041, 101.1294) -> (226.3366, 101.0767)
  line L3100 (226.3366, 101.0767) -> (226.9116, 100.9289)
  line L3101 (226.9116, 100.9289) -> (227.4628, 100.727)
  line L3102 (227.4628, 100.727) -> (227.9871, 100.4745)
  line L3103 (227.9871, 100.4745) -> (228.4818, 100.1737)
  line L3104 (228.4818, 100.1737) -> (228.9438, 99.8285)
  line L3105 (228.9438, 99.8285) -> (229.37, 99.4413)
  line L3106 (229.37, 99.4413) -> (229.7572, 99.0151)
  line L3107 (229.7572, 99.0151) -> (230.1024, 98.5532)
  line L3108 (230.1024, 98.5532) -> (230.4032, 98.0584)
  line L3109 (230.4032, 98.0584) -> (230.6557, 97.5341)
  line L3110 (230.6557, 97.5341) -> (230.8576, 96.9829)
  line L3111 (230.8576, 96.9829) -> (231.0054, 96.4079)
  line L3112 (231.0054, 96.4079) -> (231.0581, 96.1123)
  line L3113 (231.0581, 96.1123) -> (231.0963, 95.8119)
  line L3114 (231.0963, 95.8119) -> (231.1194, 95.5073)
  line L3115 (231.1194, 95.5073) -> (231.1273, 95.1987)
  line L3116 (231.1273, 95.1987) -> (231.1194, 94.8896)
  line L3117 (231.1194, 94.8896) -> (231.0963, 94.5851)
  line L3118 (231.0963, 94.5851) -> (231.0581, 94.2847)
  line L3119 (231.0581, 94.2847) -> (231.0054, 93.9894)
  line L3120 (231.0054, 93.9894) -> (230.8576, 93.4145)
  line L3121 (230.8576, 93.4145) -> (230.6557, 92.8632)
  line L3122 (230.6557, 92.8632) -> (230.4032, 92.3385)
  line L3123 (230.4032, 92.3385) -> (230.1024, 91.8438)
  line L3124 (230.1024, 91.8438) -> (229.7572, 91.3818)
  line L3125 (229.7572, 91.3818) -> (229.37, 90.956)
  line L3126 (229.37, 90.956) -> (228.9438, 90.5688)
  line L3127 (228.9438, 90.5688) -> (228.4818, 90.2233)
  line L3128 (228.4818, 90.2233) -> (227.9871, 89.9228)
  line L3129 (227.9871, 89.9228) -> (227.4628, 89.67)
  line L3130 (227.4628, 89.67) -> (226.9116, 89.4684)
  line L3131 (226.9116, 89.4684) -> (226.3366, 89.3203)
  line L3132 (226.3366, 89.3203) -> (226.041, 89.2676)
  line L3133 (226.041, 89.2676) -> (225.7406, 89.2294)
  line L3134 (225.7406, 89.2294) -> (225.436, 89.2063)
  line L3135 (225.436, 89.2063) -> (225.1273, 89.1987)
  line L3136 (225.1273, 89.1987) -> (224.8187, 89.2063)
  line L3137 (224.8187, 89.2063) -> (224.5138, 89.2294)
  line L3138 (224.5138, 89.2294) -> (224.2134, 89.2676)
  line L3139 (224.2134, 89.2676) -> (223.9181, 89.3203)
  line L3140 (223.9181, 89.3203) -> (223.3431, 89.4684)
  line L3141 (223.3431, 89.4684) -> (222.7919, 89.67)
  line L3142 (222.7919, 89.67) -> (222.2672, 89.9228)
  line L3143 (222.2672, 89.9228) -> (221.7725, 90.2233)
  line L3144 (221.7725, 90.2233) -> (221.3109, 90.5688)
  line L3145 (221.3109, 90.5688) -> (220.8847, 90.956)
  line L3146 (220.8847, 90.956) -> (220.4975, 91.3818)
  line L3147 (220.4975, 91.3818) -> (220.1519, 91.8438)
  line L3148 (220.1519, 91.8438) -> (219.8515, 92.3385)
  line L3149 (219.8515, 92.3385) -> (219.5987, 92.8632)
  line L3150 (219.5987, 92.8632) -> (219.3971, 93.4145)
  line L3151 (219.3971, 93.4145) -> (219.2493, 93.9894)
  line L3152 (219.2493, 93.9894) -> (219.1963, 94.2847)
  line L3153 (219.1963, 94.2847) -> (219.1584, 94.5851)
  line L3154 (219.1584, 94.5851) -> (219.1349, 94.8896)
  line L3155 (219.1349, 94.8896) -> (219.1274, 95.1987)
  line L3156 (204.9105, 170.452) -> (204.9336, 170.912)
  line L3157 (204.9336, 170.912) -> (205.0018, 171.3589)
  line L3158 (205.0018, 171.3589) -> (205.1127, 171.7902)
  line L3159 (205.1127, 171.7902) -> (205.264, 172.2036)
  line L3160 (205.264, 172.2036) -> (205.4538, 172.5969)
  line L3161 (205.4538, 172.5969) -> (205.6791, 172.9679)
  line L3162 (205.6791, 172.9679) -> (205.9382, 173.3143)
  line L3163 (205.9382, 173.3143) -> (206.2286, 173.634)
  line L3164 (206.2286, 173.634) -> (206.5479, 173.9244)
  line L3165 (206.5479, 173.9244) -> (206.8945, 174.1835)
  line L3166 (206.8945, 174.1835) -> (207.2656, 174.4088)
  line L3167 (207.2656, 174.4088) -> (207.659, 174.5983)
  line L3168 (207.659, 174.5983) -> (208.0724, 174.7497)
  line L3169 (208.0724, 174.7497) -> (208.5037, 174.8605)
  line L3170 (208.5037, 174.8605) -> (208.9506, 174.9287)
  line L3171 (208.9506, 174.9287) -> (209.4105, 174.9519)
  line L3172 (209.4105, 174.9519) -> (209.8707, 174.9287)
  line L3173 (209.8707, 174.9287) -> (210.3176, 174.8605)
  line L3174 (210.3176, 174.8605) -> (210.7485, 174.7497)
  line L3175 (210.7485, 174.7497) -> (211.162, 174.5983)
  line L3176 (211.162, 174.5983) -> (211.5554, 174.4088)
  line L3177 (211.5554, 174.4088) -> (211.9264, 174.1835)
  line L3178 (211.9264, 174.1835) -> (212.273, 173.9244)
  line L3179 (212.273, 173.9244) -> (212.5924, 173.634)
  line L3180 (212.5924, 173.634) -> (212.8828, 173.3143)
  line L3181 (212.8828, 173.3143) -> (213.1419, 172.9679)
  line L3182 (213.1419, 172.9679) -> (213.3675, 172.5969)
  line L3183 (213.3675, 172.5969) -> (213.557, 172.2036)
  line L3184 (213.557, 172.2036) -> (213.7082, 171.7902)
  line L3185 (213.7082, 171.7902) -> (213.8192, 171.3589)
  line L3186 (213.8192, 171.3589) -> (213.8874, 170.912)
  line L3187 (213.8874, 170.912) -> (213.9105, 170.452)
  line L3188 (213.9105, 170.452) -> (213.8874, 169.9919)
  line L3189 (213.8874, 169.9919) -> (213.8192, 169.545)
  line L3190 (213.8192, 169.545) -> (213.7082, 169.1139)
  line L3191 (213.7082, 169.1139) -> (213.557, 168.7003)
  line L3192 (213.557, 168.7003) -> (213.3675, 168.307)
  line L3193 (213.3675, 168.307) -> (213.1419, 167.936)
  line L3194 (213.1419, 167.936) -> (212.8828, 167.5896)
  line L3195 (212.8828, 167.5896) -> (212.5924, 167.2701)
  line L3196 (212.5924, 167.2701) -> (212.273, 166.9795)
  line L3197 (212.273, 166.9795) -> (211.9264, 166.7206)
  line L3198 (211.9264, 166.7206) -> (211.5554, 166.4951)
  line L3199 (211.5554, 166.4951) -> (211.162, 166.3056)
  line L3200 (211.162, 166.3056) -> (210.7485, 166.1542)
  line L3201 (210.7485, 166.1542) -> (210.3176, 166.0434)
  line L3202 (210.3176, 166.0434) -> (209.8707, 165.9752)
  line L3203 (209.8707, 165.9752) -> (209.4105, 165.952)
  line L3204 (209.4105, 165.952) -> (208.9506, 165.9752)
  line L3205 (208.9506, 165.9752) -> (208.5037, 166.0434)
  line L3206 (208.5037, 166.0434) -> (208.0724, 166.1542)
  line L3207 (208.0724, 166.1542) -> (207.659, 166.3056)
  line L3208 (207.659, 166.3056) -> (207.2656, 166.4951)
  line L3209 (207.2656, 166.4951) -> (206.8945, 166.7206)
  line L3210 (206.8945, 166.7206) -> (206.5479, 166.9795)
  line L3211 (206.5479, 166.9795) -> (206.2286, 167.2701)
  line L3212 (206.2286, 167.2701) -> (205.9382, 167.5896)
  line L3213 (205.9382, 167.5896) -> (205.6791, 167.936)
  line L3214 (205.6791, 167.936) -> (205.4538, 168.307)
  line L3215 (205.4538, 168.307) -> (205.264, 168.7003)
  line L3216 (205.264, 168.7003) -> (205.1127, 169.1139)
  line L3217 (205.1127, 169.1139) -> (205.0018, 169.545)
  line L3218 (205.0018, 169.545) -> (204.9336, 169.9919)
  line L3219 (204.9336, 169.9919) -> (204.9105, 170.452)
  line L3220 (204.9074, 126.9587) -> (204.9305, 127.4189)
  line L3221 (204.9305, 127.4189) -> (204.9987, 127.8658)
  line L3222 (204.9987, 127.8658) -> (205.1096, 128.2971)
  line L3223 (205.1096, 128.2971) -> (205.2609, 128.7105)
  line L3224 (205.2609, 128.7105) -> (205.4503, 129.1039)
  line L3225 (205.4503, 129.1039) -> (205.6756, 129.475)
  line L3226 (205.6756, 129.475) -> (205.9347, 129.8212)
  line L3227 (205.9347, 129.8212) -> (206.2251, 130.1409)
  line L3228 (206.2251, 130.1409) -> (206.5448, 130.4313)
  line L3229 (206.5448, 130.4313) -> (206.8911, 130.6904)
  line L3230 (206.8911, 130.6904) -> (207.2621, 130.9157)
  line L3231 (207.2621, 130.9157) -> (207.6555, 131.1052)
  line L3232 (207.6555, 131.1052) -> (208.069, 131.2564)
  line L3233 (208.069, 131.2564) -> (208.5003, 131.3673)
  line L3234 (208.5003, 131.3673) -> (208.9471, 131.4356)
  line L3235 (208.9471, 131.4356) -> (209.4074, 131.4586)
  line L3236 (209.4074, 131.4586) -> (209.8673, 131.4356)
  line L3237 (209.8673, 131.4356) -> (210.3141, 131.3673)
  line L3238 (210.3141, 131.3673) -> (210.7454, 131.2564)
  line L3239 (210.7454, 131.2564) -> (211.1589, 131.1052)
  line L3240 (211.1589, 131.1052) -> (211.5523, 130.9157)
  line L3241 (211.5523, 130.9157) -> (211.9233, 130.6904)
  line L3242 (211.9233, 130.6904) -> (212.2696, 130.4313)
  line L3243 (212.2696, 130.4313) -> (212.5893, 130.1409)
  line L3244 (212.5893, 130.1409) -> (212.8797, 129.8212)
  line L3245 (212.8797, 129.8212) -> (213.1388, 129.475)
  line L3246 (213.1388, 129.475) -> (213.3641, 129.1039)
  line L3247 (213.3641, 129.1039) -> (213.5535, 128.7105)
  line L3248 (213.5535, 128.7105) -> (213.7048, 128.2971)
  line L3249 (213.7048, 128.2971) -> (213.8157, 127.8658)
  line L3250 (213.8157, 127.8658) -> (213.8839, 127.4189)
  line L3251 (213.8839, 127.4189) -> (213.9074, 126.9587)
  line L3252 (213.9074, 126.9587) -> (213.8839, 126.4987)
  line L3253 (213.8839, 126.4987) -> (213.8157, 126.0519)
  line L3254 (213.8157, 126.0519) -> (213.7048, 125.6206)
  line L3255 (213.7048, 125.6206) -> (213.5535, 125.2072)
  line L3256 (213.5535, 125.2072) -> (213.3641, 124.8137)
  line L3257 (213.3641, 124.8137) -> (213.1388, 124.4427)
  line L3258 (213.1388, 124.4427) -> (212.8797, 124.0965)
  line L3259 (212.8797, 124.0965) -> (212.5893, 123.7768)
  line L3260 (212.5893, 123.7768) -> (212.2696, 123.4863)
  line L3261 (212.2696, 123.4863) -> (211.9233, 123.2273)
  line L3262 (211.9233, 123.2273) -> (211.5523, 123.002)
  line L3263 (211.5523, 123.002) -> (211.1589, 122.8125)
  line L3264 (211.1589, 122.8125) -> (210.7454, 122.6612)
  line L3265 (210.7454, 122.6612) -> (210.3141, 122.5503)
  line L3266 (210.3141, 122.5503) -> (209.8673, 122.4821)
  line L3267 (209.8673, 122.4821) -> (209.4074, 122.4587)
  line L3268 (209.4074, 122.4587) -> (208.9471, 122.4821)
  line L3269 (208.9471, 122.4821) -> (208.5003, 122.5503)
  line L3270 (208.5003, 122.5503) -> (208.069, 122.6612)
  line L3271 (208.069, 122.6612) -> (207.6555, 122.8125)
  line L3272 (207.6555, 122.8125) -> (207.2621, 123.002)
  line L3273 (207.2621, 123.002) -> (206.8911, 123.2273)
  line L3274 (206.8911, 123.2273) -> (206.5448, 123.4863)
  line L3275 (206.5448, 123.4863) -> (206.2251, 123.7768)
  line L3276 (206.2251, 123.7768) -> (205.9347, 124.0965)
  line L3277 (205.9347, 124.0965) -> (205.6756, 124.4427)
  line L3278 (205.6756, 124.4427) -> (205.4503, 124.8137)
  line L3279 (205.4503, 124.8137) -> (205.2609, 125.2072)
  line L3280 (205.2609, 125.2072) -> (205.1096, 125.6206)
  line L3281 (205.1096, 125.6206) -> (204.9987, 126.0519)
  line L3282 (204.9987, 126.0519) -> (204.9305, 126.4987)
  line L3283 (204.9305, 126.4987) -> (204.9074, 126.9587)
  line L3284 (239.0948, 199.2139) -> (239.1065, 199.677)
  line L3285 (239.1065, 199.677) -> (239.1413, 200.134)
  line L3286 (239.1413, 200.134) -> (239.1985, 200.5845)
  line L3287 (239.1985, 200.5845) -> (239.2777, 201.0277)
  line L3288 (239.2777, 201.0277) -> (239.378, 201.463)
  line L3289 (239.378, 201.463) -> (239.4992, 201.8902)
  line L3290 (239.4992, 201.8902) -> (239.6408, 202.3084)
  line L3291 (239.6408, 202.3084) -> (239.8021, 202.717)
  line L3292 (239.8021, 202.717) -> (239.9823, 203.1158)
  line L3293 (239.9823, 203.1158) -> (240.181, 203.5039)
  line L3294 (240.181, 203.5039) -> (240.3977, 203.8808)
  line L3295 (240.3977, 203.8808) -> (240.632, 204.2458)
  line L3296 (240.632, 204.2458) -> (240.8828, 204.5987)
  line L3297 (240.8828, 204.5987) -> (241.1498, 204.9387)
  line L3298 (241.1498, 204.9387) -> (241.433, 205.2652)
  line L3299 (241.433, 205.2652) -> (241.7306, 205.5778)
  line L3300 (241.7306, 205.5778) -> (242.0435, 205.8758)
  line L3301 (242.0435, 205.8758) -> (242.37, 206.1586)
  line L3302 (242.37, 206.1586) -> (242.7101, 206.4258)
  line L3303 (242.7101, 206.4258) -> (243.0629, 206.6768)
  line L3304 (243.0629, 206.6768) -> (243.428, 206.9109)
  line L3305 (243.428, 206.9109) -> (243.8049, 207.1276)
  line L3306 (243.8049, 207.1276) -> (244.1928, 207.3264)
  line L3307 (244.1928, 207.3264) -> (244.5914, 207.5065)
  line L3308 (244.5914, 207.5065) -> (245.0004, 207.6678)
  line L3309 (245.0004, 207.6678) -> (245.4186, 207.8092)
  line L3310 (245.4186, 207.8092) -> (245.8455, 207.9305)
  line L3311 (245.8455, 207.9305) -> (246.2809, 208.0311)
  line L3312 (246.2809, 208.0311) -> (246.7243, 208.1101)
  line L3313 (246.7243, 208.1101) -> (247.1746, 208.1673)
  line L3314 (247.1746, 208.1673) -> (247.6317, 208.2021)
  line L3315 (247.6317, 208.2021) -> (248.0948, 208.2138)
  line L3316 (248.0948, 208.2138) -> (248.5578, 208.2021)
  line L3317 (248.5578, 208.2021) -> (249.0149, 208.1673)
  line L3318 (249.0149, 208.1673) -> (249.4656, 208.1101)
  line L3319 (249.4656, 208.1101) -> (249.9086, 208.0311)
  line L3320 (249.9086, 208.0311) -> (250.3441, 207.9305)
  line L3321 (250.3441, 207.9305) -> (250.7713, 207.8092)
  line L3322 (250.7713, 207.8092) -> (251.1891, 207.6678)
  line L3323 (251.1891, 207.6678) -> (251.5981, 207.5065)
  line L3324 (251.5981, 207.5065) -> (251.9967, 207.3264)
  line L3325 (251.9967, 207.3264) -> (252.3846, 207.1276)
  line L3326 (252.3846, 207.1276) -> (252.7615, 206.9109)
  line L3327 (252.7615, 206.9109) -> (253.1267, 206.6768)
  line L3328 (253.1267, 206.6768) -> (253.4798, 206.4258)
  line L3329 (253.4798, 206.4258) -> (253.8195, 206.1586)
  line L3330 (253.8195, 206.1586) -> (254.1461, 205.8758)
  line L3331 (254.1461, 205.8758) -> (254.4589, 205.5778)
  line L3332 (254.4589, 205.5778) -> (254.7569, 205.2652)
  line L3333 (254.7569, 205.2652) -> (255.0397, 204.9387)
  line L3334 (255.0397, 204.9387) -> (255.3067, 204.5987)
  line L3335 (255.3067, 204.5987) -> (255.5579, 204.2458)
  line L3336 (255.5579, 204.2458) -> (255.7918, 203.8808)
  line L3337 (255.7918, 203.8808) -> (256.0085, 203.5039)
  line L3338 (256.0085, 203.5039) -> (256.2073, 203.1158)
  line L3339 (256.2073, 203.1158) -> (256.3875, 202.717)
  line L3340 (256.3875, 202.717) -> (256.5487, 202.3084)
  line L3341 (256.5487, 202.3084) -> (256.6903, 201.8902)
  line L3342 (256.6903, 201.8902) -> (256.8115, 201.463)
  line L3343 (256.8115, 201.463) -> (256.9118, 201.0277)
  line L3344 (256.9118, 201.0277) -> (256.991, 200.5845)
  line L3345 (256.991, 200.5845) -> (257.0482, 200.134)
  line L3346 (257.0482, 200.134) -> (257.083, 199.677)
  line L3347 (257.083, 199.677) -> (257.0947, 199.2139)
  line L3348 (257.0947, 199.2139) -> (257.083, 198.7507)
  line L3349 (257.083, 198.7507) -> (257.0482, 198.2937)
  line L3350 (257.0482, 198.2937) -> (256.991, 197.8432)
  line L3351 (256.991, 197.8432) -> (256.9118, 197.4)
  line L3352 (256.9118, 197.4) -> (256.8115, 196.9645)
  line L3353 (256.8115, 196.9645) -> (256.6903, 196.5375)
  line L3354 (256.6903, 196.5375) -> (256.5487, 196.1193)
  line L3355 (256.5487, 196.1193) -> (256.3875, 195.7107)
  line L3356 (256.3875, 195.7107) -> (256.2073, 195.3119)
  line L3357 (256.2073, 195.3119) -> (256.0085, 194.9238)
  line L3358 (256.0085, 194.9238) -> (255.7918, 194.547)
  line L3359 (255.7918, 194.547) -> (255.5579, 194.1818)
  line L3360 (255.5579, 194.1818) -> (255.3067, 193.829)
  line L3361 (255.3067, 193.829) -> (255.0397, 193.489)
  line L3362 (255.0397, 193.489) -> (254.7569, 193.1624)
  line L3363 (254.7569, 193.1624) -> (254.4589, 192.8499)
  line L3364 (254.4589, 192.8499) -> (254.1461, 192.5519)
  line L3365 (254.1461, 192.5519) -> (253.8195, 192.2691)
  line L3366 (253.8195, 192.2691) -> (253.4798, 192.0019)
  line L3367 (253.4798, 192.0019) -> (253.1267, 191.7509)
  line L3368 (253.1267, 191.7509) -> (252.7615, 191.5168)
  line L3369 (252.7615, 191.5168) -> (252.3846, 191.3001)
  line L3370 (252.3846, 191.3001) -> (251.9967, 191.1013)
  line L3371 (251.9967, 191.1013) -> (251.5981, 190.9212)
  line L3372 (251.5981, 190.9212) -> (251.1891, 190.7599)
  line L3373 (251.1891, 190.7599) -> (250.7713, 190.6185)
  line L3374 (250.7713, 190.6185) -> (250.3441, 190.4972)
  line L3375 (250.3441, 190.4972) -> (249.9086, 190.3966)
  line L3376 (249.9086, 190.3966) -> (249.4656, 190.3176)
  line L3377 (249.4656, 190.3176) -> (249.0149, 190.2602)
  line L3378 (249.0149, 190.2602) -> (248.5578, 190.2256)
  line L3379 (248.5578, 190.2256) -> (248.0948, 190.2139)
  line L3380 (248.0948, 190.2139) -> (247.6317, 190.2256)
  line L3381 (247.6317, 190.2256) -> (247.1746, 190.2602)